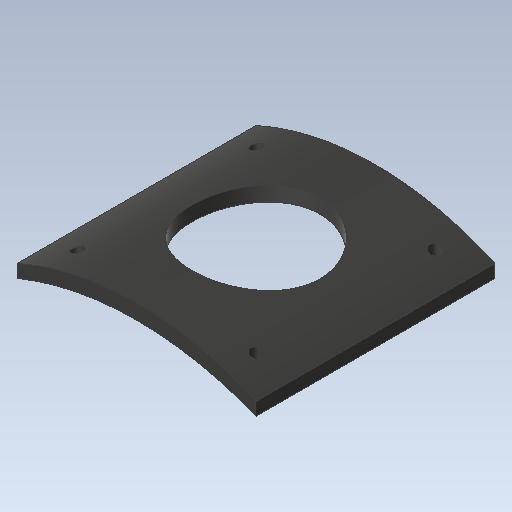
# Autodesk Inventor part: dopasowywacz
Saved by Autodesk Inventor 2020 (Build 240168000, 168)
## iProperties
Created: 2019-06-01
Part Number: dopasowywacz
Material: ABS Plastic
Document SubType Name: Modeling
Designer: Esterka
Density: 1.06 g/cm^3
Appearance: Smooth - White
Author: Esterka
Autodesk Inventor part; units mm, degrees
ref_plane "YZ Plane" through (0, 0, 0) normal (1, 0, 0) x (0, 1, 0)
ref_plane "XY Plane" through (0, 0, 0) normal (0, 0, 1) x (1, 0, 0)
sketch "Sketch1" plane through (0, 0, 0) normal (0, 0, 1) x (1, 0, 0)
  arc A0 (85.0917, -2.3076) -> (-9.9083, -2.3076) centre (37.5917, -117.9309) ccw
  arc A1 (85.0917, 2.8037) -> (-9.9083, 2.8037) centre (37.5917, -101.9281) ccw
  line L0 (-9.9083, -2.3076) -> (-9.9083, 2.8037)
  line L1 (85.0917, -2.3076) -> (85.0917, 2.8037)
  point P0 (0, 0)
  constraints: 4 end point, 4 point on circle, 2 centre point
extrude "Extrusion1" add sketch "Sketch1" along normal blind 95
sketch "Sketch2" plane through (0, 0, 0) normal (0, 1, 0) x (-1, 0, 0)
  line L0 (12.4083, 0) -> (12.4083, 95) projected
  line L1 (-85.0917, 95) -> (9.9083, 95) projected
  line L2 (9.9083, 0) -> (-85.0917, 0) projected
  line L3 (-87.5917, 0) -> (-87.5917, 95) projected
  line L4 (9.9083, 0) -> (9.9083, 95) projected
  line L5 (-85.0917, 0) -> (-85.0917, 95) projected
  point P0 (0, 0)
  point P1 (-2.0917, 83)
  point P2 (-2.0917, 12)
  point P3 (-73.0917, 12)
  point P4 (-73.0917, 83)
  dimension "d14" = 12
  dimension "d30" = 12
  dimension "d31" = 12
  dimension "d32" = 12
  dimension "d33" = 12
  dimension "d34" = 12
  dimension "d35" = 12
  dimension "d37" = 12
  constraints: 2 other
  measures "d14" distance from line of L1 point (-73.092, 83)
  measures "d30" distance from line of point (-2.092, 12) L2
  measures "d31" distance from line of L4 point (-2.092, 12)
  measures "d32" distance from line of L4 point (-2.092, 83)
  measures "d33" distance from line of L5 point (-73.092, 12)
  measures "d34" distance from line of L2 point (-73.092, 12)
  measures "d35" distance from line of L5 point (-73.092, 83)
  measures "d37" distance from line of L1 point (-2.092, 83)
ref_plane "Work Plane1" through (0, 15, 0) normal (0, 1, 0) x (-1, 0, 0)
sketch "Sketch3" plane through (0, 15, 0) normal (0, 1, 0) x (-1, 0, 0)
  point P0 (0, 0)
  point P1 (-2.0917, 12)
  point P2 (-2.0917, 83)
  point P3 (-73.0917, 83)
  point P4 (-73.0917, 12)
hole "Hole1" at (73.0917, 15, 83) at (2.0917, 15, 83) at (2.0917, 15, 12) at (73.0917, 15, 12) direction (0, -1, 0) diameter 4.5 depth 34.9875 tip angle 118 clearance for "Countersunk Flat Head Screw ISO 2009/7046" size "M4" standard "ISO"
sketch "Sketch4" plane through (0, 15, 0) normal (0, 1, 0) x (-1, 0, 0)
  line L0 (9.9083, 0) -> (-85.0917, 0) projected
  circle A0 centre (-37.5917, 47.5) radius 25.4
  line L1 (-85.0917, 0) -> (-85.0917, 95) projected
  point P0 (0, 0)
  dimension "d23" = 47.5
  dimension "d25" = 50.8
  dimension "d36" = 47.5
  constraints: 1 centre point, 1 coincident
  measures "d23" distance from line of L0 point (-37.592, 47.5)
  measures "d25" diameter of A0
  measures "d36" distance from line of L1 point (-37.592, 47.5)
extrude "Extrusion2" cut sketch "Sketch4" against normal blind 24.2875
body "Solid1"
